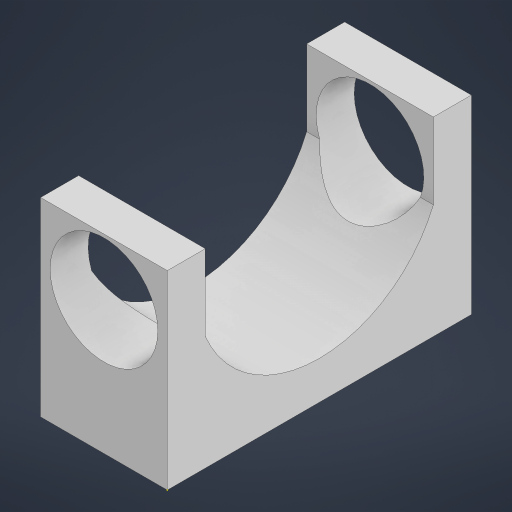
# Autodesk Inventor part: Part4
Saved by Autodesk Inventor 2023 (Build 270158030, 158C)
## iProperties
Created: 2023-02-03
Part Number: Part4
Material: Generic
Document SubType Name: Modeling
Designer: Monster
Density: 1 g/cm^3
Appearance: Default
Author: Monster
Autodesk Inventor part; units mm, degrees
ref_plane "YZ Plane" through (0, 0, 0) normal (1, 0, 0) x (0, 1, 0)
ref_plane "XZ Plane" through (0, 0, 0) normal (0, 1, 0) x (-1, 0, 0)
ref_plane "XY Plane" through (0, 0, 0) normal (0, 0, 1) x (1, 0, 0)
sketch "Sketch1" plane through (0, 0, 0) normal (0, 0, 1) x (1, 0, 0)
  point P0 (0, 0)
sketch "Sketch2" plane through (0, 0, 0) normal (0, 1, 0) x (-1, 0, 0)
  line L0 (0, 0) -> (0, -24)
  line L1 (0, -24) -> (10, -24)
  line L2 (10, -24) -> (10, 0)
  line L3 (10, 0) -> (0, 0)
  dimension "d0" = 24
  dimension "d1" = 10
  constraints: 8 end point, 3 perpendicular, 1 vertical
  measures "d0" distance of L0.start L0.end
  measures "d1" distance of L0.end L1.end
extrude "Extrusion1" add sketch "Sketch2" along normal blind 15
sketch "Sketch5" plane through (0, 0, 0) normal (1, 0, 0) x (0, 0, -1)
  line L0 (0, 0) -> (24, 0) projected
  line L1 (24, 0) -> (24, 15) projected
  line L2 (0, 15) -> (24, 15) projected
  line L3 (0, 0) -> (0, 15) projected
  line L4 (24, 15) -> (0, 15) projected
  line L5 (0, 15) -> (3, 15)
  line L6 (24, 15) -> (21, 15)
  line L7 (24, 0) -> (0, 0) projected
  line L8 (12, 0) -> (12, 3)
  line L9 (3, 15) -> (3, 9)
  line L10 (3, 9) -> (21, 9)
  line L11 (21, 9) -> (21, 15)
  arc A0 (3, 9) -> (21, 9) centre (12, 12.75) ccw
  dimension "d4" = 3
  dimension "d5" = 3
  dimension "d7" = 3
  dimension "d8" = 6
  constraints: 12 end point, 3 point on circle, 2 perpendicular, 2 point on line, 2 vertical, 1 centre point, 1 midpoint
  measures "d4" distance of L2.start L5.end
  measures "d5" distance of L1.end L6.end
  measures "d7" distance of L8.start L8.end
  measures "d8" distance of L5.end L9.end
extrude "Extrusion2" cut sketch "Sketch5" against normal blind 17 contours A0 L10 | L2 L11 L10 L9
sketch "Sketch6" plane through (-10, 0, 0) normal (0, 0, 1) x (1, 0, 0)
  line L0 (0, 0) -> (10, 0) projected
  line L1 (10, 0) -> (10, 15) projected
  line L2 (0, 15) -> (10, 15) projected
  line L3 (0, 0) -> (0, 15) projected
  line L4 (0, 15) -> (10, 15) projected
  line L5 (5, 15) -> (5, 10.5)
  circle A0 centre (5, 10.5) radius 4.25
  dimension "d11" = 4.5
  dimension "d12" = 8.5
  constraints: 2 end point, 1 centre point, 1 coincident, 1 midpoint, 1 vertical
  measures "d11" distance of L5.start L5.end
  measures "d12" diameter of A0
extrude "Extrusion3" cut sketch "Sketch6" against normal blind 31.25 contours A0
body "Solid1"
